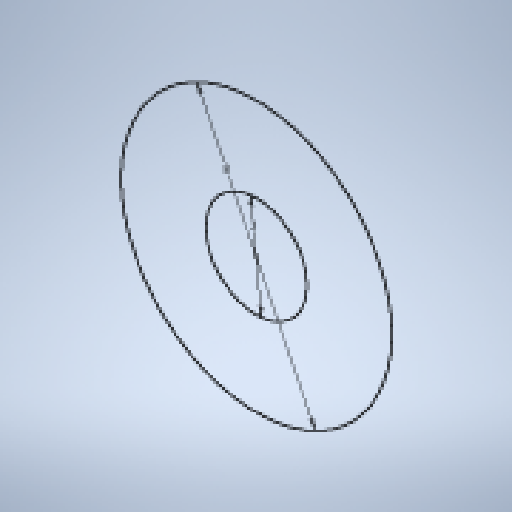
# Autodesk Inventor part: Cam - Lever
Saved by Autodesk Inventor 2023.2 (Build 272271000, 271)
## iProperties
Created: 2024-01-19
Part Number: Cam - Lever
Material: Nylon 6/6
Document SubType Name: Modeling
Designer: Nathan Cai
Density: 1.13 g/cm^3
Appearance: Nylon 6
Author: Nathan Cai
Autodesk Inventor part; units mm, degrees
ref_plane "YZ Plane" through (0, 0, 0) normal (1, 0, 0) x (0, 1, 0)
ref_plane "XZ Plane" through (0, 0, 0) normal (0, 1, 0) x (-1, 0, 0)
ref_plane "XY Plane" through (0, 0, 0) normal (0, 0, 1) x (1, 0, 0)
sketch "Sketch1" plane through (0, 0, 0) normal (0, 0, 1) x (1, 0, 0)
  circle A0 centre (0, 0) radius 1.5
  circle A1 centre (0, 0) radius 4
  circle A2 centre (0, 0) radius 7 construction
  line L0 (0, 0) -> (0, 7) construction
  circle A3 centre (-1, 13.3125) radius 6.35
  line L1 (0, 0) -> (0, 7) construction
  line L2 (4, 0) -> (4, 7)
  line L3 (-4, 7) -> (-4, 0)
  arc A4 (-4, 0) -> (4, 0) centre (0, 0) ccw
  arc A5 (4, 7) -> (-4, 7) centre (0, 7) ccw
  point P0 (0, 3.5)
  point P1 (-3.9251, 7.7702)
  point P2 (4, 0)
  point P3 (3.5364, 8.8691)
  point P4 (-4, 0)
  point P5 (-3.941, 7.6846)
  dimension "d2" = 14
  dimension "d0" = 3
  dimension "d1" = 8
  dimension "d3" = 12.7
  dimension "d4" = 4
  dimension "d9" = 1
  constraints: 10 end point, 5 centre point, 5 point on circle, 4 tangent, 3 coincident, 2 equal length, 1 midpoint, 1 vertical, 1 vertical alignment, 3 other
  measures "d0" diameter of A0
  measures "d1" diameter of A1
  measures "d3" diameter of A3
  measures "d4" radius of A5
  measures "d9" distance from line of L0 A3.centre
extrude "Extrusion1" add sketch "Sketch1" along normal blind 4.7625 contours A1 | A1 L3 A5 A3 L2
fillet "Fillet1" radius 1.5 2 edges at (3.5364, 8.8691, 2.3813) (-3.941, 7.6846, 2.3813)
sketch "Sketch2" plane through (0, 0, 0) normal (0, 0, -1) x (-1, 0, 0)
  arc A0 (4, 5.6071) -> (2.2134, 7.0795) centre (2.5, 5.6071) ccw projected
  arc A1 (-1.8312, 7.6286) -> (2.2134, 7.0795) centre (1, 13.3125) ccw projected
  arc A2 (-1.8312, 7.6286) -> (-4, 6.2859) centre (-2.5, 6.2859) ccw projected
  line L0 (-4, 0) -> (-4, 6.2859) projected
  arc A3 (-4, 0) -> (4, 0) centre (0, 0) ccw projected
  line L1 (4, 5.6071) -> (4, 0) projected
  circle A4 centre (0, 0) radius 1.5 projected
  circle A5 centre (0, 0) radius 8.2648 construction
  constraints: 1 centre point, 1 coincident, 1 tangent
equation "\"d4\" = 0.5 * d1"
body "Solid1"
